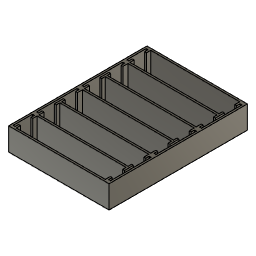
Battery Case (6X-AAA-Single) (Autodesk Fusion 360 design; units mm, degrees)
Autodesk Fusion 360 part; units mm, degrees
sketch "Base" plane through (0, 0, 0) normal (0, 0, 1) x (1, 0, 0) in component "6X-AAA-Single"
  line L0 (26.5, -36.5) -> (-26.5, -36.5)
  line L1 (-26.5, -36.5) -> (-26.5, 36.5)
  line L2 (-26.5, 36.5) -> (26.5, 36.5)
  line L3 (26.5, 36.5) -> (26.5, -36.5)
  line L4 (26.5, -36.5) -> (-26.5, 36.5) construction
  line L5 (-26.5, -36.5) -> (26.5, 36.5) construction
  line L6 (25.5, -35.5) -> (-25.5, -35.5)
  line L7 (-25.5, -35.5) -> (-25.5, 35.5)
  line L8 (-25.5, 35.5) -> (25.5, 35.5)
  line L9 (25.5, 35.5) -> (25.5, -35.5)
  line L10 (0, 35.5) -> (0, -35.5) construction
  line L11 (-25.5, 0) -> (25.5, 0) construction
  line L12 (-25.5, 12) -> (25.5, 12) construction
  line L13 (-25.5, 24) -> (25.5, 24) construction
  line L14 (-25.5, -12) -> (25.5, -12) construction
  line L15 (-25.5, -24) -> (25.5, -24) construction
  line L16 (-25.5, -35.5) -> (-24.5, -35.5)
  line L17 (-24.5, -35.5) -> (-24.5, -35.1)
  line L18 (-24.5, -35.1) -> (-25.5, -35.1)
  line L19 (-25.5, -35.1) -> (-25.5, -35.5)
  line L20 (-24.5, -35.5) -> (-23.5, -35.5)
  line L21 (-23.5, -35.5) -> (-23.5, -33.25)
  line L22 (-23.5, -33.25) -> (-24.5, -33.25)
  line L23 (-24.5, -33.25) -> (-24.5, -35.5)
  line L24 (-25.5, 35.5) -> (-24.5, 35.5)
  line L25 (-24.5, 35.5) -> (-24.5, 35.1)
  line L26 (-24.5, 35.1) -> (-25.5, 35.1)
  line L27 (-25.5, 35.1) -> (-25.5, 35.5)
  line L28 (-24.5, 35.5) -> (-23.5, 35.5)
  line L29 (-23.5, 35.5) -> (-23.5, 33.25)
  line L30 (-23.5, 33.25) -> (-24.5, 33.25)
  line L31 (-24.5, 33.25) -> (-24.5, 35.5)
  line L32 (-25, 35.1) -> (-25, -35.1) construction
  line L33 (-24, -33.25) -> (-24, 33.25) construction
  line L34 (25.5, -35.5) -> (24.5, -35.5)
  line L35 (24.5, -35.5) -> (24.5, -34.7)
  line L36 (24.5, -34.7) -> (25.5, -34.7)
  line L37 (25.5, -34.7) -> (25.5, -35.5)
  line L38 (24.5, -35.5) -> (23.5, -35.5)
  line L39 (23.5, -35.5) -> (23.5, -32.85)
  line L40 (23.5, -32.85) -> (24.5, -32.85)
  line L41 (24.5, -32.85) -> (24.5, -35.5)
  line L42 (25.5, 35.5) -> (24.5, 35.5)
  line L43 (24.5, 35.5) -> (24.5, 34.7)
  line L44 (24.5, 34.7) -> (25.5, 34.7)
  line L45 (25.5, 34.7) -> (25.5, 35.5)
  line L46 (24.5, 35.5) -> (23.5, 35.5)
  line L47 (23.5, 35.5) -> (23.5, 32.85)
  line L48 (23.5, 32.85) -> (24.5, 32.85)
  line L49 (24.5, 32.85) -> (24.5, 35.5)
  line L50 (25, 34.7) -> (25, -34.7) construction
  line L51 (24, -32.85) -> (24, 32.85) construction
  line L52 (-23.5, -26.75) -> (-24.5, -26.75)
  line L53 (-24.5, -26.75) -> (-24.5, -21.25)
  line L54 (-24.5, -21.25) -> (-23.5, -21.25)
  line L55 (-23.5, -21.25) -> (-23.5, -26.75)
  line L56 (-23.5, -26.75) -> (-24.5, -21.25) construction
  line L57 (-24.5, -26.75) -> (-23.5, -21.25) construction
  line L58 (-24.5, -24.9) -> (-25.5, -24.9)
  line L59 (-25.5, -24.9) -> (-25.5, -23.1)
  line L60 (-25.5, -23.1) -> (-24.5, -23.1)
  line L61 (-24.5, -23.1) -> (-24.5, -24.9)
  line L62 (-24.5, -24.9) -> (-25.5, -23.1) construction
  line L63 (-25.5, -24.9) -> (-24.5, -23.1) construction
  line L64 (-25.5, -22.7) -> (-24.5, -22.7)
  line L65 (-24.5, -20.85) -> (-23.5, -20.85)
  line L66 (24.5, -26.35) -> (23.5, -26.35)
  line L67 (23.5, -26.35) -> (23.5, -21.65)
  line L68 (23.5, -21.65) -> (24.5, -21.65)
  line L69 (24.5, -21.65) -> (24.5, -26.35)
  line L70 (24.5, -26.35) -> (23.5, -21.65) construction
  line L71 (23.5, -26.35) -> (24.5, -21.65) construction
  line L72 (-25.5, -22.7) -> (-25.5, -23.1)
  line L73 (-24.5, -22.7) -> (-24.5, -23.1)
  line L74 (-24.5, -20.85) -> (-24.5, -21.25)
  line L75 (-23.5, -20.85) -> (-23.5, -21.25)
  line L76 (23.5, -24.5) -> (-23.5, -24.5)
  line L77 (-23.5, -24.5) -> (-23.5, -23.5)
  line L78 (-23.5, -23.5) -> (23.5, -23.5)
  line L79 (23.5, -23.5) -> (23.5, -24.5)
  line L80 (23.5, -24.5) -> (-23.5, -23.5) construction
  line L81 (-23.5, -24.5) -> (23.5, -23.5) construction
  line L82 (-23.5, -9.65) -> (-24.5, -9.65)
  line L83 (-24.5, -9.65) -> (-24.5, -14.35)
  line L84 (-24.5, -14.35) -> (-23.5, -14.35)
  line L85 (-23.5, -14.35) -> (-23.5, -9.65)
  line L86 (-23.5, -9.65) -> (-24.5, -14.35) construction
  line L87 (-24.5, -9.65) -> (-23.5, -14.35) construction
  line L88 (24.5, -15.15) -> (23.5, -15.15)
  line L89 (23.5, -15.15) -> (23.5, -8.85)
  line L90 (23.5, -8.85) -> (24.5, -8.85)
  line L91 (24.5, -8.85) -> (24.5, -15.15)
  line L92 (24.5, -15.15) -> (23.5, -8.85) construction
  line L93 (23.5, -15.15) -> (24.5, -8.85) construction
  line L94 (25.5, -13.3) -> (24.5, -13.3)
  line L95 (24.5, -13.3) -> (24.5, -10.7)
  line L96 (24.5, -10.7) -> (25.5, -10.7)
  line L97 (25.5, -10.7) -> (25.5, -13.3)
  line L98 (25.5, -13.3) -> (24.5, -10.7) construction
  line L99 (24.5, -13.3) -> (25.5, -10.7) construction
  line L100 (23.5, -12.5) -> (-23.5, -12.5)
  line L101 (-23.5, -12.5) -> (-23.5, -11.5)
  line L102 (-23.5, -11.5) -> (23.5, -11.5)
  line L103 (23.5, -11.5) -> (23.5, -12.5)
  line L104 (23.5, -12.5) -> (-23.5, -11.5) construction
  line L105 (-23.5, -12.5) -> (23.5, -11.5) construction
  line L106 (-23.5, -3.15) -> (-24.5, -3.15)
  line L107 (-24.5, -3.15) -> (-24.5, 3.15)
  line L108 (-24.5, 3.15) -> (-23.5, 3.15)
  line L109 (-23.5, 3.15) -> (-23.5, -3.15)
  line L110 (-23.5, -3.15) -> (-24.5, 3.15) construction
  line L111 (-24.5, -3.15) -> (-23.5, 3.15) construction
  line L112 (-24.5, -1.3) -> (-25.5, -1.3)
  line L113 (-25.5, -1.3) -> (-25.5, 1.3)
  line L114 (-25.5, 1.3) -> (-24.5, 1.3)
  line L115 (-24.5, 1.3) -> (-24.5, -1.3)
  line L116 (-24.5, -1.3) -> (-25.5, 1.3) construction
  line L117 (-25.5, -1.3) -> (-24.5, 1.3) construction
  line L118 (24.5, -2.35) -> (23.5, -2.35)
  line L119 (23.5, -2.35) -> (23.5, 2.35)
  line L120 (23.5, 2.35) -> (24.5, 2.35)
  line L121 (24.5, 2.35) -> (24.5, -2.35)
  line L122 (24.5, -2.35) -> (23.5, 2.35) construction
  line L123 (23.5, -2.35) -> (24.5, 2.35) construction
  line L124 (23.5, -0.5) -> (-23.5, -0.5)
  line L125 (-23.5, -0.5) -> (-23.5, 0.5)
  line L126 (-23.5, 0.5) -> (23.5, 0.5)
  line L127 (23.5, 0.5) -> (23.5, -0.5)
  line L128 (23.5, -0.5) -> (-23.5, 0.5) construction
  line L129 (-23.5, -0.5) -> (23.5, 0.5) construction
  line L130 (24.5, 8.85) -> (23.5, 8.85)
  line L131 (23.5, 8.85) -> (23.5, 15.15)
  line L132 (23.5, 15.15) -> (24.5, 15.15)
  line L133 (24.5, 15.15) -> (24.5, 8.85)
  line L134 (24.5, 8.85) -> (23.5, 15.15) construction
  line L135 (23.5, 8.85) -> (24.5, 15.15) construction
  line L136 (25.5, 10.7) -> (24.5, 10.7)
  line L137 (24.5, 10.7) -> (24.5, 13.3)
  line L138 (24.5, 13.3) -> (25.5, 13.3)
  line L139 (25.5, 13.3) -> (25.5, 10.7)
  line L140 (25.5, 10.7) -> (24.5, 13.3) construction
  line L141 (24.5, 10.7) -> (25.5, 13.3) construction
  line L142 (-23.5, 9.65) -> (-24.5, 9.65)
  line L143 (-24.5, 9.65) -> (-24.5, 14.35)
  line L144 (-24.5, 14.35) -> (-23.5, 14.35)
  line L145 (-23.5, 14.35) -> (-23.5, 9.65)
  line L146 (-23.5, 9.65) -> (-24.5, 14.35) construction
  line L147 (-24.5, 9.65) -> (-23.5, 14.35) construction
  line L148 (23.5, 11.5) -> (-23.5, 11.5)
  line L149 (-23.5, 11.5) -> (-23.5, 12.5)
  line L150 (-23.5, 12.5) -> (23.5, 12.5)
  line L151 (23.5, 12.5) -> (23.5, 11.5)
  line L152 (23.5, 11.5) -> (-23.5, 12.5) construction
  line L153 (-23.5, 11.5) -> (23.5, 12.5) construction
  line L154 (24.5, 21.65) -> (23.5, 21.65)
  line L155 (23.5, 21.65) -> (23.5, 26.35)
  line L156 (23.5, 26.35) -> (24.5, 26.35)
  line L157 (24.5, 26.35) -> (24.5, 21.65)
  line L158 (24.5, 21.65) -> (23.5, 26.35) construction
  line L159 (23.5, 21.65) -> (24.5, 26.35) construction
  line L160 (-23.5, 26.75) -> (-24.5, 26.75)
  line L161 (-24.5, 26.75) -> (-24.5, 21.25)
  line L162 (-24.5, 21.25) -> (-23.5, 21.25)
  line L163 (-23.5, 21.25) -> (-23.5, 26.75)
  line L164 (-23.5, 26.75) -> (-24.5, 21.25) construction
  line L165 (-24.5, 26.75) -> (-23.5, 21.25) construction
  line L166 (-24.5, 23.1) -> (-25.5, 23.1)
  line L167 (-25.5, 23.1) -> (-25.5, 24.9)
  line L168 (-25.5, 24.9) -> (-24.5, 24.9)
  line L169 (-24.5, 24.9) -> (-24.5, 23.1)
  line L170 (-24.5, 23.1) -> (-25.5, 24.9) construction
  line L171 (-25.5, 23.1) -> (-24.5, 24.9) construction
  line L172 (-24.5, 22.7) -> (-25.5, 22.7)
  line L173 (-24.5, 20.85) -> (-23.5, 20.85)
  line L174 (-25.5, 23.1) -> (-25.5, 22.7)
  line L175 (-24.5, 23.1) -> (-24.5, 22.7)
  line L176 (-24.5, 21.25) -> (-24.5, 20.85)
  line L177 (-23.5, 21.25) -> (-23.5, 20.85)
  line L178 (23.5, 24.5) -> (-23.5, 24.5)
  line L179 (-23.5, 24.5) -> (-23.5, 23.5)
  line L180 (-23.5, 23.5) -> (23.5, 23.5)
  line L181 (23.5, 23.5) -> (23.5, 24.5)
  line L182 (23.5, 24.5) -> (-23.5, 23.5) construction
  line L183 (-23.5, 24.5) -> (23.5, 23.5) construction
  line L184 (-23.5, 33.25) -> (-23.5, 26.75)
  line L185 (-23.5, 20.85) -> (-23.5, 14.35)
  line L186 (-23.5, 9.65) -> (-23.5, 3.15)
  line L187 (-23.5, -3.15) -> (-23.5, -9.65)
  line L188 (-23.5, -14.35) -> (-23.5, -20.85)
  line L189 (-23.5, -26.75) -> (-23.5, -33.25)
  line L190 (23.5, -26.35) -> (23.5, -32.85)
  line L191 (23.5, -15.15) -> (23.5, -21.65)
  line L192 (23.5, -2.35) -> (23.5, -8.85)
  line L193 (23.5, 8.85) -> (23.5, 2.35)
  line L194 (23.5, 21.65) -> (23.5, 15.15)
  line L195 (23.5, 32.85) -> (23.5, 26.35)
  point P0 (-24, -24)
  point P1 (-25, -24)
  point P2 (24, -24)
  point P3 (0, -24)
  point P4 (-24, -12)
  point P5 (24, -12)
  point P6 (25, -12)
  point P7 (0, -12)
  point P8 (-24, 0)
  point P9 (-25, 0)
  point P10 (24, 0)
  point P11 (24, 12)
  point P12 (25, 12)
  point P13 (-24, 12)
  point P14 (0, 12)
  point P15 (24, 24)
  point P16 (-24, 24)
  point P17 (-25, 24)
  point P18 (0, 24)
  dimension "d1" = 53
  dimension "d2" = 73
  dimension "d3" = 1
  dimension "d7" = 12
  dimension "d9" = 12
  dimension "d11" = 12
  dimension "d12" = 12
  dimension "d14" = 1
  dimension "d15" = 0.4
  dimension "d16" = 1
  dimension "d17" = 2.25
  dimension "d18" = 1
  dimension "d19" = 0.4
  dimension "d20" = 1
  dimension "d21" = 2.25
  dimension "d22" = 1
  dimension "d23" = 0.8
  dimension "d24" = 1
  dimension "d25" = 2.65
  dimension "d26" = 1
  dimension "d27" = 0.8
  dimension "d28" = 1
  dimension "d29" = 2.65
  dimension "d30" = 1
  dimension "d31" = 5.5
  dimension "d32" = 1
  dimension "d33" = 1.8
  dimension "d34" = -0.4
  dimension "d35" = -0.4
  dimension "d36" = 1
  dimension "d37" = 4.7
  dimension "d38" = 47
  dimension "d39" = 1
  dimension "d40" = 1
  dimension "d41" = 4.7
  dimension "d42" = 1
  dimension "d43" = 6.3
  dimension "d44" = 1
  dimension "d45" = 2.6
  dimension "d46" = 47
  dimension "d47" = 1
  dimension "d48" = 1
  dimension "d49" = 6.3
  dimension "d50" = 1
  dimension "d51" = 2.6
  dimension "d52" = 1
  dimension "d53" = 4.7
  dimension "d54" = 47
  dimension "d55" = 1
  dimension "d56" = 1
  dimension "d57" = 6.3
  dimension "d58" = 1
  dimension "d59" = 2.6
  dimension "d60" = 1
  dimension "d61" = 4.7
  dimension "d62" = 47
  dimension "d63" = 1
  dimension "d64" = 1
  dimension "d65" = 4.7
  dimension "d66" = 1
  dimension "d67" = 5.5
  dimension "d68" = 1
  dimension "d69" = 1.8
  dimension "d70" = -0.4
  dimension "d71" = 0.4
  dimension "d72" = 47
  dimension "d73" = 1
  constraint horizontal L0
  constraint perpendicular L0 L1
  constraint parallel L0 L2
  constraint parallel L1 L3
  constraint coincident L4 origin
  constraint coincident L5 origin
  constraint midpoint L8 L10.start
  constraint midpoint L6 L10.end
  constraint midpoint L7 L11.start
  constraint midpoint L9 L11.end
  constraint coincident L7 L12.start
  constraint coincident L9 L12.end
  constraint perpendicular L9 L12
  constraint coincident L7 L13.start
  constraint coincident L9 L13.end
  constraint perpendicular L9 L13
  constraint coincident L7 L14.start
  constraint coincident L9 L14.end
  constraint perpendicular L9 L14
  constraint coincident L7 L15.start
  constraint perpendicular L10 L15
  constraint horizontal L16
  constraint vertical L17
  constraint horizontal L18
  constraint vertical L19
  constraint horizontal L20
  constraint vertical L21
  constraint horizontal L22
  constraint vertical L23
  constraint horizontal L24
  constraint vertical L25
  constraint horizontal L26
  constraint vertical L27
  constraint horizontal L28
  constraint vertical L29
  constraint horizontal L30
  constraint vertical L31
  constraint midpoint L26 L32.start
  constraint midpoint L18 L32.end
  constraint midpoint L22 L33.start
  constraint perpendicular L15 L33
  constraint midpoint L30 L33.end
  constraint horizontal L34
  constraint vertical L35
  constraint horizontal L36
  constraint vertical L37
  constraint horizontal L38
  constraint vertical L39
  constraint horizontal L40
  constraint vertical L41
  constraint horizontal L42
  constraint vertical L43
  constraint horizontal L44
  constraint vertical L45
  constraint horizontal L46
  constraint vertical L47
  constraint horizontal L48
  constraint vertical L49
  constraint midpoint L44 L50.start
  constraint midpoint L36 L50.end
  constraint midpoint L40 L51.start
  constraint midpoint L48 L51.end
  constraint horizontal L52
  constraint perpendicular L52 L53
  constraint parallel L52 L54
  constraint parallel L53 L55
  constraint coincident L56 P0
  constraint coincident L57 P0
  constraint coincident L15 P0
  constraint coincident L33 P0
  constraint horizontal L58
  constraint perpendicular L58 L59
  constraint parallel L58 L60
  constraint parallel L59 L61
  constraint coincident L62 P1
  constraint coincident L63 P1
  constraint coincident L15 P1
  constraint coincident L32 P1
  constraint horizontal L66
  constraint perpendicular L66 L67
  constraint parallel L66 L68
  constraint parallel L67 L69
  constraint coincident L70 P2
  constraint coincident L71 P2
  constraint coincident L15 P2
  constraint coincident L51 P2
  constraint perpendicular L60 L72
  constraint perpendicular L60 L73
  constraint perpendicular L54 L75
  constraint horizontal L76
  constraint perpendicular L76 L77
  constraint parallel L76 L78
  constraint parallel L77 L79
  constraint coincident L80 P3
  constraint coincident L81 P3
  constraint midpoint L15 P3
  constraint horizontal L82
  constraint perpendicular L82 L83
  constraint parallel L82 L84
  constraint parallel L83 L85
  constraint coincident L86 P4
  constraint coincident L87 P4
  constraint coincident L14 P4
  constraint coincident L33 P4
  constraint horizontal L88
  constraint perpendicular L88 L89
  constraint parallel L88 L90
  constraint parallel L89 L91
  constraint coincident L92 P5
  constraint coincident L93 P5
  constraint coincident L51 P5
  constraint coincident L14 P5
  constraint horizontal L94
  constraint perpendicular L94 L95
  constraint parallel L94 L96
  constraint parallel L95 L97
  constraint coincident L98 P6
  constraint coincident L99 P6
  constraint coincident L14 P6
  constraint coincident L50 P6
  constraint horizontal L100
  constraint perpendicular L100 L101
  constraint parallel L100 L102
  constraint parallel L101 L103
  constraint coincident L104 P7
  constraint coincident L105 P7
  constraint midpoint L14 P7
  constraint horizontal L106
  constraint perpendicular L106 L107
  constraint parallel L106 L108
  constraint parallel L107 L109
  constraint coincident L110 P8
  constraint coincident L111 P8
  constraint coincident L11 P8
  constraint coincident L33 P8
  constraint horizontal L112
  constraint perpendicular L112 L113
  constraint parallel L112 L114
  constraint parallel L113 L115
  constraint coincident L116 P9
  constraint coincident L117 P9
  constraint midpoint L32 P9
  constraint horizontal L118
  constraint perpendicular L118 L119
  constraint parallel L118 L120
  constraint parallel L119 L121
  constraint coincident L122 P10
  constraint coincident L123 P10
  constraint midpoint L51 P10
  constraint horizontal L124
  constraint perpendicular L124 L125
  constraint parallel L124 L126
  constraint parallel L125 L127
  constraint coincident L128 origin
  constraint coincident L129 origin
  constraint horizontal L130
  constraint perpendicular L130 L131
  constraint parallel L130 L132
  constraint parallel L131 L133
  constraint coincident L134 P11
  constraint coincident L135 P11
  constraint coincident L12 P11
  constraint coincident L51 P11
  constraint horizontal L136
  constraint perpendicular L136 L137
  constraint parallel L136 L138
  constraint parallel L137 L139
  constraint coincident L140 P12
  constraint coincident L141 P12
  constraint coincident L12 P12
  constraint coincident L50 P12
  constraint horizontal L142
  constraint perpendicular L142 L143
  constraint parallel L142 L144
  constraint parallel L143 L145
  constraint coincident L146 P13
  constraint coincident L147 P13
  constraint coincident L12 P13
  constraint coincident L33 P13
  constraint horizontal L148
  constraint perpendicular L148 L149
  constraint parallel L148 L150
  constraint parallel L149 L151
  constraint coincident L152 P14
  constraint coincident L153 P14
  constraint midpoint L12 P14
  constraint horizontal L154
  constraint perpendicular L154 L155
  constraint parallel L154 L156
  constraint parallel L155 L157
  constraint coincident L158 P15
  constraint coincident L159 P15
  constraint coincident L13 P15
  constraint coincident L51 P15
  constraint horizontal L160
  constraint perpendicular L160 L161
  constraint parallel L160 L162
  constraint parallel L161 L163
  constraint coincident L164 P16
  constraint coincident L165 P16
  constraint coincident L13 P16
  constraint coincident L33 P16
  constraint horizontal L166
  constraint perpendicular L166 L167
  constraint parallel L166 L168
  constraint parallel L167 L169
  constraint coincident L170 P17
  constraint coincident L171 P17
  constraint coincident L13 P17
  constraint coincident L32 P17
  constraint horizontal L178
  constraint perpendicular L178 L179
  constraint parallel L178 L180
  constraint parallel L179 L181
  constraint coincident L182 P18
  constraint coincident L183 P18
  constraint midpoint L13 P18
  constraint perpendicular L144 L185
  measures "d1" distance of L1.end L2.end
  measures "d2" distance of L0.end L1.end
  measures "d7" distance of L12 L13
  measures "d9" distance of L11 L12
  measures "d11" distance of L11 L14
  measures "d12" distance of L14 L15
  measures "d14" distance of L6.end L16.end
  measures "d15" distance of L6.end L18.end
  measures "d16" distance of L16.end L20.end
  measures "d17" distance of L16.end L22.end
  measures "d18" distance of L7.end L24.end
  measures "d19" distance of L7.end L26.end
  measures "d20" distance of L24.end L28.end
  measures "d21" distance of L24.end L30.end
  measures "d22" distance of L6.start L34.end
  measures "d23" distance of L6.start L36.end
  measures "d24" distance of L34.end L38.end
  measures "d25" distance of L34.end L40.end
  measures "d26" distance of L8.end L42.end
  measures "d27" distance of L8.end L44.end
  measures "d28" distance of L42.end L46.end
  measures "d29" distance of L42.end L48.end
  measures "d30" distance of L53.end L54.end
  measures "d31" distance of L52.end L53.end
  measures "d32" distance of L59.end L60.end
  measures "d33" distance of L58.end L59.end
  measures "d36" distance of L67.end L68.end
  measures "d37" distance of L66.end L67.end
  measures "d38" distance of L77.end L78.end
  measures "d39" distance of L76.end L77.end
  measures "d40" distance of L83.end L84.end
  measures "d41" distance of L82.end L83.end
  measures "d42" distance of L89.end L90.end
  measures "d43" distance of L88.end L89.end
  measures "d44" distance of L95.end L96.end
  measures "d45" distance of L94.end L95.end
  measures "d46" distance of L101.end L102.end
  measures "d47" distance of L100.end L101.end
  measures "d48" distance of L107.end L108.end
  measures "d49" distance of L106.end L107.end
  measures "d50" distance of L113.end L114.end
  measures "d51" distance of L112.end L113.end
  measures "d52" distance of L119.end L120.end
  measures "d53" distance of L118.end L119.end
  measures "d54" distance of L125.end L126.end
  measures "d55" distance of L124.end L125.end
  measures "d56" distance of L131.end L132.end
  measures "d57" distance of L130.end L131.end
  measures "d58" distance of L137.end L138.end
  measures "d59" distance of L136.end L137.end
  measures "d60" distance of L143.end L144.end
  measures "d61" distance of L142.end L143.end
  measures "d62" distance of L149.end L150.end
  measures "d63" distance of L148.end L149.end
  measures "d64" distance of L155.end L156.end
  measures "d65" distance of L154.end L155.end
  measures "d66" distance of L161.end L162.end
  measures "d67" distance of L160.end L161.end
  measures "d68" distance of L167.end L168.end
  measures "d69" distance of L166.end L167.end
  measures "d72" distance of L179.end L180.end
  measures "d73" distance of L178.end L179.end
extrude "Extrude1" add sketch "Base" along normal blind 12 contours L0 L1 L2 L3 | L6 L9 L34 L35 L36 L37 L41 | L6 L35 L38 L39 L40 L41 | L9 L91 L94 L95 L96 L97 | L6 L17 L20 L21 L22 L23 | L88 L89 L90 L91 L95 L103 | L6 L7 L16 L17 L18 L19 L23 | L66 L67 L68 L69 L79 | L9 L133 L136 L137 L138 L139 | L52 L53 L54 L55 L61 L73 L77 | L55 L67 L76 L77 L78 L79 | L130 L131 L132 L133 L137 L151 | L8 L9 L42 L43 L44 L45 L49 | L85 L89 L100 L101 L102 L103 | L7 L53 L58 L59 L60 L61 | L8 L43 L46 L47 L48 L49 | L118 L119 L120 L121 L127 | L82 L83 L84 L85 L101 | L7 L53 L60 L64 L72 L73 | L54 L65 L74 L75 | L131 L145 L148 L149 L150 L151 | L109 L119 L124 L125 L126 L127 | L154 L155 L156 L157 L181 | L142 L143 L144 L145 L149 | L106 L107 L108 L109 L115 L125 | L7 L107 L112 L113 L114 L115 | L8 L25 L28 L29 L30 L31 | L155 L163 L178 L179 L180 L181 | L7 L8 L24 L25 L26 L27 L31 | L160 L161 L162 L163 L169 L175 L179 | L7 L161 L166 L172 L174 L175 | L162 L173 L176 L177 | L7 L161 L166 L167 L168 L169 in component "6X-AAA-Single"
extrude "Extrude2" add sketch "Base" along normal blind 1.5 contours L9 L36 L40 L41 L66 L68 L69 L88 L91 L94 L190 L191 | L9 L90 L91 L96 L118 L120 L121 L130 L133 L136 L192 L193 | L7 L18 L22 L23 L52 L53 L58 L189 | L9 L44 L48 L49 L132 L133 L138 L154 L156 L157 L194 L195 | L7 L53 L64 L65 L74 L82 L83 L84 L106 L107 L112 L187 L188 | L7 L107 L108 L114 L142 L143 L144 L161 L172 L173 L176 L185 L186 | L7 L26 L30 L31 L160 L161 L168 L184 in component "6X-AAA-Single"
extrude "Extrude3" add sketch "Base" along normal blind 1 contours L6 L21 L39 L55 L67 L76 L189 L190 | L55 L67 L75 L78 L85 L89 L100 L188 L191 | L85 L89 L102 L109 L119 L124 L187 L192 | L109 L119 L126 L131 L145 L148 L186 L193 | L131 L145 L150 L155 L163 L177 L180 L185 L194 | L8 L29 L47 L155 L163 L178 L184 L195 in component "6X-AAA-Single"
component "6X-AAA-Single" placed x (1, 0, 0) y (0, 1, 0) z (0, 0, 1) at (0, 0, 0)
named bodies: "6X-AAA-Single"
